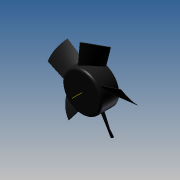
# Autodesk Inventor part: fan
Saved by Autodesk Inventor 2014 (Build 180170000, 170)
## iProperties
Shininess: 64.0
Angle Display Precision: 2
Document Length Units: 11272
Document Angle Units: 11279
Document Time Units: 11290
Document Mass Units: 11286
Document Length Units Precision: 3
Document Angle Units Precision: 2
Created: 2001-12-19
Part Number: fan
Document SubType Name: Modeling
Designer: Administrator
Density: 1 g/cm^3
Material: Generic
Appearance: Glossy - Black
Density: 0.0
Volumn: 0.0
Area: 0.0
PropertySet Name: Model Information
Control State: 0
Master: False
Checked Out: False
Author: Administrator
Autodesk Inventor part; units mm, degrees
sketch "Sketch1" plane through (0, 0, 0) normal (0, 0, 1) x (1, 0, 0)
  circle A0 centre (146.7584, -19.9786) radius 28.8925
  dimension "d0" = 57.785
  constraints: 1 centre point
  measures "d0" diameter of A0
extrude "Extrusion1" add sketch "Sketch1" along normal blind 26.416
fillet "Fillet1" radius 3.175 1 edges at (117.8659, -19.9786, 26.416)
sketch "Sketch2" plane through (146.7584, -19.9786, 26.416) normal (0, 0, 1) x (1, 0, 0)
  circle A0 centre (0, 0) radius 25.7175 projected
  circle A1 centre (0, 0) radius 28.8925 projected
  line L0 (0, 0) -> (0, 28.8925)
  constraints: 2 end point, 1 vertical, 1 vertical alignment, 1 other
ref_plane "Work Plane1" through (146.7584, 8.9139, 26.416) normal (0, 1, 0) x (-1, 0, 0)
ref_plane "Work Plane2" through (146.7584, 47.0139, 26.416) normal (0, 1, 0) x (-1, 0, 0)
sketch "Sketch4" plane through (146.7584, 47.0139, 26.416) normal (0, 1, 0) x (-1, 0, 0)
  arc A0 (8.5086, -7.0723) -> (-20.8007, -25.463) centre (26.2475, -67.8935) ccw
  arc A1 (8.7479, -7.7998) -> (8.5086, -7.0723) centre (8.6159, -7.4401) ccw
  arc A2 (8.7479, -7.7998) -> (-20.1726, -25.4365) centre (38.7405, -89.5113) ccw
  arc A3 (-20.8007, -25.463) -> (-20.1726, -25.4365) centre (-20.5023, -25.0779) ccw
  constraints: 8 point on circle, 4 centre point, 3 tangent
ref_plane "Work Plane3" through (146.7584, -3.7861, 26.416) normal (0, 1, 0) x (-1, 0, 0)
sketch "Sketch5" plane through (146.7584, -3.7861, 26.416) normal (0, 1, 0) x (-1, 0, 0)
  arc A0 (10.3547, -4.2858) -> (-8.7274, -24.7268) centre (37.7816, -49.0164) ccw
  arc A1 (10.9013, -5.1233) -> (10.3547, -4.2858) centre (10.6161, -4.7122) ccw
  arc A2 (10.9013, -5.1233) -> (-8.2354, -24.7103) centre (52.0982, -64.5149) ccw
  arc A3 (-8.7274, -24.7268) -> (-8.2354, -24.7103) centre (-8.4873, -24.5442) ccw
  constraints: 8 point on circle, 4 centre point, 3 tangent
loft "Loft1" add profiles "Sketch5", "Sketch4"
pattern_circular "Circular Pattern1" count 5 over 360 about axis through (146.7584, -19.9786, 0) along (0, 0, 1) of "Loft1"
sketch "Sketch6" plane through (146.7584, -19.9786, 26.416) normal (0, 0, 1) x (1, 0, 0)
  circle A0 centre (0, 0) radius 25.7175 projected
  circle A1 centre (0, 0) radius 57.15
  circle A2 centre (0, 1.4745) radius 74.4601
  dimension "d11" = 114.3
  constraints: 2 centre point, 1 coincident
  measures "d11" diameter of A1
extrude "Extrusion2" cut sketch "Sketch6" against normal through all contours A2
sketch "Sketch7" plane through (146.7584, -19.9786, 0) normal (0, 0, -1) x (-1, 0, 0)
  circle A0 centre (0, 0) radius 28.8925 projected
  circle A1 centre (0, 0) radius 27.6225
  dimension "d17" = 1.27
  constraints: 1 centre point, 1 coincident
  measures "d17" radial gap between concentric circles of A0 A1
extrude "Extrusion3" cut sketch "Sketch7" against normal blind 22.225 contours A1
body "Solid1"
